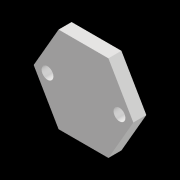
# Autodesk Inventor part: EncoderBoard
Saved by Autodesk Inventor 2020 (Build 240168000, 168)
## iProperties
Created: 2021-02-20
Part Number: EncoderBoard
Material: Generic
Document SubType Name: Modeling
Designer: valer
Density: 1 g/cm^3
Appearance: Default
Author: valer
Autodesk Inventor part; units mm, degrees
ref_plane "YZ Plane" through (0, 0, 0) normal (1, 0, 0) x (0, 1, 0)
ref_plane "XZ Plane" through (0, 0, 0) normal (0, 1, 0) x (-1, 0, 0)
ref_plane "XY Plane" through (0, 0, 0) normal (0, 0, 1) x (1, 0, 0)
sketch "Sketch1" plane through (0, 0, 0) normal (0, 0, 1) x (1, 0, 0)
  line L0 (-3.9, 2.4325) -> (3.9, 2.4325) construction
  line L1 (3.9, 2.4325) -> (3.9, -2.4325) construction
  line L2 (3.9, -2.4325) -> (-3.9, -2.4325) construction
  line L3 (-3.9, -2.4325) -> (-3.9, 2.4325) construction
  line L4 (-3.9, 2.4325) -> (3.9, -2.4325) construction
  line L5 (3.9, 2.4325) -> (-3.9, -2.4325) construction
  circle A0 centre (0, 0) radius 0.5 construction
  line L6 (-20.447, 0) -> (20.447, 0) construction
  line L7 (6.3025, 10.9163) -> (12.605, 0)
  line L8 (12.605, 0) -> (6.3025, -10.9163)
  line L9 (6.3025, -10.9163) -> (-6.3025, -10.9163)
  line L10 (-6.3025, -10.9163) -> (-12.605, 0)
  line L11 (-12.605, 0) -> (-6.3025, 10.9163)
  line L12 (-6.3025, 10.9163) -> (6.3025, 10.9163)
  circle A1 centre (-9.105, 0) radius 1.5
  circle A2 centre (9.105, 0) radius 1.5
  point P0 (0, 10.9163)
  dimension "d0" = 7.8
  dimension "d1" = 4.865
  dimension "d2" = 1
  dimension "d3" = 0
  dimension "d7" = 3
  dimension "d8" = 3.5
  dimension "d9" = 21.8325
  dimension "d10" = 8.4838
  dimension "d11" = 10.9162
  dimension "d12" = 10.9162
  dimension "d13" = 10.9162
  dimension "d14" = 3.9
  dimension "d15" = 6.7914
  dimension "d16" = 3.0311
  dimension "d17" = 3.0311
  dimension "d18" = 10.9162
  dimension "d19" = 28.6239
  constraints: 26 end point, 4 parallel, 3 centre point, 3 midpoint, 1 coincident, 1 equal radius, 1 horizontal, 1 perpendicular, 1 point on line, 13 other
  measures "d0" distance of L3.end L0.end
  measures "d1" distance of L3.start L3.end
  measures "d2" diameter of A0
  measures "d3" distance from line of point (0, 0) L6
  measures "d7" diameter of A1
  measures "d8" distance of L10.end A1.centre
  measures "d9" distance between parallel lines of L7 L10
  measures "d10" distance between parallel lines of L12 L0
  measures "d11" distance between parallel lines of L6 L12
  measures "d12" distance from line of point (0, 0) L7
  measures "d13" distance from line of point (0, 0) L8
  measures "d14" distance from line of point (0, 0) L1
  measures "d15" distance from line of L6.end L7
  measures "d16" distance from line of A2.centre L7
  measures "d17" distance from line of A2.centre L8
  measures "d18" distance from line of point (0, 0) L7
  measures "d19" distance from line of L6.start L7
extrude "Extrusion1" add sketch "Sketch1" along normal blind 3.3
body "Solid1"
